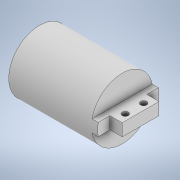
# Autodesk Inventor part: drive_shaft_v3
Saved by Autodesk Inventor 2022 (Build 260153000, 153)
## iProperties
Created: 2022-05-21
Part Number: drive_shaft_v3
Material: Generic
Document SubType Name: Modeling
Designer: kylem
Density: 1 g/cm^3
Appearance: Default
Author: kylem
Autodesk Inventor part; units mm, degrees
ref_plane "YZ Plane" through (0, 0, 0) normal (1, 0, 0) x (0, 1, 0)
ref_plane "XZ Plane" through (0, 0, 0) normal (0, 1, 0) x (-1, 0, 0)
sketch "Sketch1" plane through (0, 0, 0) normal (0, 1, 0) x (-1, 0, 0)
  line L0 (0, 0) -> (20, 0)
  line L1 (20, 0) -> (20, -2)
  line L2 (20, -2) -> (0, -2)
  line L3 (0, -2) -> (0, 0)
  dimension "d0" = 20
  dimension "d1" = 2
  constraints: 8 end point, 2 parallel, 1 horizontal, 1 perpendicular
  measures "d0" distance of L1.end L2.end
  measures "d1" distance of L0.end L1.end
extrude "Extrusion1" add sketch "Sketch1" along normal blind 2
sketch "Sketch2" plane through (0, 2, 0) normal (0, 1, 0) x (1, 0, 0)
  line L0 (0, 2) -> (-20, 2) projected
  line L1 (0, 2) -> (0, 4)
  line L2 (0, 4) -> (2, 4)
  line L3 (2, 4) -> (2, -2)
  line L4 (2, -2) -> (0, -2)
  line L5 (0, 0) -> (0, 2) projected
  line L6 (0, -2) -> (0, 0)
  dimension "d4" = 2
  dimension "d5" = 2
  dimension "d6" = 6
  constraints: 10 end point, 3 perpendicular, 1 collinear, 1 point on line, 1 vertical
  measures "d4" distance of L0.start L1.end
  measures "d5" distance of L1.end L2.end
  measures "d6" distance of L2.end L3.end
extrude "Extrusion2" add sketch "Sketch2" against normal blind 2
sketch "Sketch3" plane through (0, 2, 0) normal (0, 1, 0) x (1, 0, 0)
  line L0 (0, 0) -> (0, -2) projected
  line L1 (0, -2) -> (0, -1)
  line L2 (2, 4) -> (2, -2) projected
  line L3 (2, -2) -> (2, -0.5)
  line L4 (2, -0.5) -> (1, -0.5)
  circle A0 centre (1, -0.5) radius 0.5
  line L5 (2, 1) -> (1.5, 1)
  circle A1 centre (1, 2.5) radius 0.5
  dimension "d9" = 1.5
  dimension "d10" = 1
  dimension "d11" = 1
  constraints: 8 end point, 2 centre point, 2 midpoint, 1 coincident, 1 horizontal, 1 perpendicular, 1 point on line, 1 symmetric about line, 1 other
  measures "d9" distance of L2.end L3.end
  measures "d10" distance of L3.end L4.end
  measures "d11" diameter of A0
extrude "Extrusion3" cut sketch "Sketch3" against normal blind 2
sketch "Sketch4" plane through (0, 2, -4) normal (-1, 0, 0) x (0, 0, 1)
  line L0 (2, 0) -> (4, 0) projected
  line L1 (3, 0) -> (3, -2)
  line L2 (2, -2) -> (4, -2) projected
  circle A0 centre (3, -1) radius 1
  line L3 (2, -2) -> (2, 0) projected
  circle A1 centre (3, -1) radius 1.4142
  constraints: 3 midpoint, 2 end point, 1 centre point, 1 coincident, 1 tangent, 3 other
extrude "Extrusion4" cut sketch "Sketch4" along normal blind 100 contours L0 A0 L3 | L3 A1 | L0 A1 L2 A0 | A0 L2 L3
ref_plane "Work Plane1" through (-14, 1, -1) normal (-1, 0, 0) x (0, 0, 1)
sketch "Sketch5" plane through (-14, 1, -1) normal (-1, 0, 0) x (0, 0, 1)
  circle A0 centre (0, 0) radius 5
  point P0 (1, -1)
  dimension "d17" = 10
  constraints: 1 centre point
  measures "d17" diameter of A0
extrude "Extrusion5" add sketch "Sketch5" along normal mid plane 1
sketch "Sketch6" plane through (-20, 1, -1) normal (-1, 0, 0) x (0, 0, 1)
  circle A0 centre (0, 0) radius 5
  point P0 (1, -1)
  constraints: 1 centre point
extrude "Extrusion6" cut sketch "Sketch6" against normal blind 5.5
sketch "Sketch7" plane through (-13.5, 1, -1) normal (1, 0, 0) x (0, 0, -1)
  circle A0 centre (0, 0) radius 5 projected
  circle A1 centre (0, 0) radius 5
  point P0 (-1, -1)
  constraints: 1 centre point, 1 coincident
extrude "Extrusion7" add sketch "Sketch7" along normal blind 13.5
sketch "Sketch8" plane through (0, 0, 0) normal (0, -1, 0) x (1, 0, 0)
  line L0 (2, -4) -> (-1, -4)
  line L1 (-1, -4) -> (-1, -6.7389)
  line L2 (-1, -6.7389) -> (2, -6.7389)
  line L3 (2, -6.7389) -> (2, -4)
  line L4 (2, -4) -> (2, 2) projected
  line L5 (2, 2) -> (-1, 2)
  line L6 (-1, 2) -> (-1, 5.2785)
  line L7 (-1, 5.2785) -> (2, 5.2785)
  line L8 (2, 5.2785) -> (2, 2)
  line L9 (2, 5.2785) -> (-1, 5.2785)
  line L10 (-1, 5.2785) -> (-1, -6.7389)
  line L11 (-1, -6.7389) -> (2, -6.7389)
  line L12 (2, -6.7389) -> (2, 5.2785)
  point P0 (0, 0)
  dimension "d24" = 3
  dimension "d25" = 3
  constraints: 24 end point, 6 parallel, 3 horizontal, 3 perpendicular
  measures "d24" distance of L2.end L1.end
  measures "d25" distance of L6.end L7.end
extrude "Extrusion8" cut sketch "Sketch8" along normal blind 13.5
ref_plane "Work Plane2" through (0, 1, 0) normal (0, -1, 0) x (1, 0, 0)
mirror "Mirror1" about plane through (0, 1, 0) normal (0, -1, 0) of "Extrusion8"
body "Solid1"
